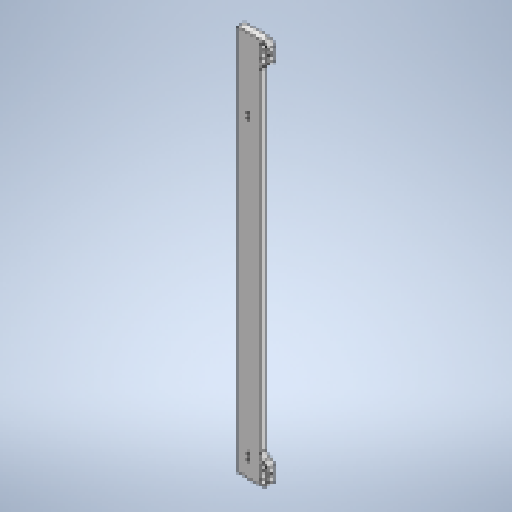
# Autodesk Inventor part: VerticalSlideMiddle2.1
Saved by Autodesk Inventor 2023 (Build 270158000, 158)
## iProperties
Created: 2022-10-14
Part Number: VerticalSlideMiddle2.1
Material: Generic
Document SubType Name: Modeling
Designer: deli
Density: 1 g/cm^3
Appearance: Default
Author: deli
Autodesk Inventor part; units mm, degrees
ref_plane "YZ Plane" through (0, 0, 0) normal (1, 0, 0) x (0, 1, 0)
ref_plane "XZ Plane" through (0, 0, 0) normal (0, 1, 0) x (-1, 0, 0)
ref_plane "XY Plane" through (0, 0, 0) normal (0, 0, 1) x (1, 0, 0)
sketch "Sketch1" plane through (0, 0, 0) normal (0, 0, 1) x (1, 0, 0)
  line L0 (-59.8946, 167.5645) -> (-83.1446, 167.5645)
  line L1 (-83.1446, 167.5645) -> (-83.1446, -185.4355)
  line L2 (-83.1446, -185.4355) -> (-59.8946, -185.4355)
  circle A0 centre (-73.1446, -170.4355) radius 1.25
  circle A1 centre (-73.1446, 99.5645) radius 1.25
  circle A2 centre (-73.1446, -165.9355) radius 1.25
  circle A3 centre (-73.1446, 104.0645) radius 1.25
  arc A4 (-57.6446, 163.3145) -> (-62.1446, 163.3145) centre (-59.8946, 163.3145) ccw
  arc A5 (-62.1446, 151.3145) -> (-57.6446, 151.3145) centre (-59.8946, 151.3145) ccw
  line L3 (-57.6446, 163.3145) -> (-57.6446, 151.3145)
  line L4 (-62.1446, 151.3145) -> (-62.1446, 163.3145)
  line L5 (-55.6446, 163.3145) -> (-55.6446, 151.3145)
  arc A6 (-55.6446, 163.3145) -> (-59.8946, 167.5645) centre (-59.8946, 163.3145) ccw
  arc A7 (-59.3946, 147.094) -> (-63.1446, 142.8736) centre (-58.8946, 142.8736) ccw
  arc A8 (-59.3946, 147.094) -> (-55.6446, 151.3145) centre (-59.8946, 151.3145) ccw
  arc A9 (-62.1446, -181.1855) -> (-57.6446, -181.1855) centre (-59.8946, -181.1855) ccw
  arc A10 (-57.6446, -169.1855) -> (-62.1446, -169.1855) centre (-59.8946, -169.1855) ccw
  line L6 (-57.6446, -169.1855) -> (-57.6446, -181.1855)
  line L7 (-62.1446, -169.1855) -> (-62.1446, -181.1855)
  line L8 (-55.6446, -169.1855) -> (-55.6446, -181.1855)
  arc A11 (-59.8946, -185.4355) -> (-55.6446, -181.1855) centre (-59.8946, -181.1855) ccw
  arc A12 (-63.1446, -160.7445) -> (-59.3946, -164.965) centre (-58.8946, -160.7445) ccw
  line L9 (-63.1446, -160.7445) -> (-63.1446, 142.8736)
  arc A13 (-55.6446, -169.1855) -> (-59.3946, -164.965) centre (-59.8946, -169.1855) ccw
  point P0 (0, 0)
  dimension "d1" = 353
  dimension "d2" = 2.5
  dimension "d3" = 10
  dimension "d4" = 15
  dimension "d9" = 10
  dimension "d10" = 10
  dimension "d11" = 2
  dimension "d12" = 270
  dimension "d13" = 10
  dimension "d14" = 2
  dimension "d15" = 4.5
  dimension "d17" = 12
  dimension "d20" = 2
  dimension "d22" = 12
  dimension "d24" = 1
  dimension "d25" = 1
  constraints: 22 point on circle, 20 end point, 16 tangent, 14 centre point, 10 equal radius, 5 parallel, 4 coincident, 2 point on line, 2 vertical, 1 horizontal, 1 perpendicular
  measures "d1" distance of L1.end L0.end
  measures "d2" diameter of A0
  measures "d3" distance from line of L1 A0.centre
  measures "d4" distance from line of L2 A0.centre
  measures "d9" distance from line of L1 A1.centre
  measures "d10" distance from line of L1 A2.centre
  measures "d12" distance of A1.centre A0.centre
  measures "d13" distance from line of L1 A3.centre
  measures "d15" diameter of A4
  measures "d17" distance of A5.centre A4.centre
  measures "d20" radial gap between concentric circles of A4 A6
  measures "d22" distance of A9.centre A10.centre
  measures "d24" distance between parallel lines of L9 L7
  measures "d25" distance between parallel lines of L4 L9
extrude "Extrusion1" add sketch "Sketch1" along normal blind 6.35
sketch "Sketch2" plane through (-55.6446, 151.3145, 0) normal (1, 0, 0) x (0, 0, -1)
  line L0 (0, 0) -> (0, 12) construction
  line L1 (0, 12) -> (-6.35, 12) construction
  line L2 (-6.35, 0) -> (-6.35, 12) construction
  line L3 (0, 0) -> (-6.35, 0) construction
  line L4 (0, -332.5) -> (0, -320.5) construction
  line L5 (0, -320.5) -> (-6.35, -320.5) construction
  line L6 (-6.35, -332.5) -> (-6.35, -320.5) construction
  line L7 (0, -332.5) -> (-6.35, -332.5) construction
  line L8 (-6.35, 12) -> (0, 0) construction
  line L9 (-6.35, 0) -> (0, 12) construction
  circle A0 centre (-3.175, 6) radius 1.25
  line L10 (-6.35, -320.5) -> (0, -332.5) construction
  line L11 (-6.35, -332.5) -> (0, -320.5) construction
  circle A1 centre (-3.175, -326.5) radius 1.25
  point P0 (0, -151.3145)
  dimension "d28" = 2.5
  constraints: 8 end point, 2 centre point, 2 midpoint, 1 equal radius
  measures "d28" diameter of A0
extrude "Extrusion2" cut sketch "Sketch2" against normal blind 17
thread "Thread1" size "M3x0.5" class "6H" standard "ANSI Metric M Profile" full length
thread "Thread2" size "M3x0.5" class "6H" standard "ANSI Metric M Profile" full length
thread "Thread3" size "M3x0.5" class "6H" standard "ANSI Metric M Profile" full length
thread "Thread4" size "M3x0.5" class "6H" standard "ANSI Metric M Profile" full length
thread "Thread5" size "M3x0.5" class "6H" standard "ANSI Metric M Profile" full length
thread "Thread6" size "M3x0.5" class "6H" standard "ANSI Metric M Profile" full length
equation "\"d3\" = 0.5 * d23"
equation "\"d9\" = d3"
equation "\"d10\" = d3"
equation "\"d13\" = d9"
equation "\"d14\" = d11"
equation "\"d22\" = d17"
equation "\"d24\" = d25"
equation "\"d23\" = 20"
body "Solid1"
